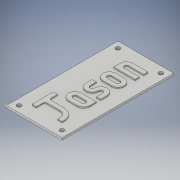
# Autodesk Inventor part: JASON
Saved by Autodesk Inventor 2017 (Build 210142000, 142)
## iProperties
Created: 2016-09-21
Part Number: JASON
Material: Generic
Document SubType Name: Modeling
Designer: vslabsal
Density: 1 g/cm^3
Appearance: Default
Author: vslabsal
Autodesk Inventor part; units mm, degrees
ref_plane "YZ Plane" through (0, 0, 0) normal (1, 0, 0) x (0, 1, 0)
ref_plane "XZ Plane" through (0, 0, 0) normal (0, 1, 0) x (-1, 0, 0)
ref_plane "XY Plane" through (0, 0, 0) normal (0, 0, 1) x (1, 0, 0)
sketch "Sketch1" plane through (0, 0, 0) normal (0, 1, 0) x (-1, 0, 0)
  line L0 (-82.55, -165.1) -> (0, -165.1)
  line L1 (0, -165.1) -> (0, 0)
  line L2 (0, 0) -> (-82.55, 0)
  line L3 (-82.55, 0) -> (-82.55, -165.1)
  circle A0 centre (-73.025, -155.575) radius 3.175
  circle A1 centre (-73.025, -155.575) radius 3.175
  circle A2 centre (-9.525, -155.575) radius 3.175
  circle A3 centre (-9.525, -155.575) radius 3.175
  circle A4 centre (-73.025, -9.525) radius 3.175
  circle A5 centre (-73.025, -9.525) radius 3.175
  circle A6 centre (-9.525, -9.525) radius 3.175
  circle A7 centre (-9.525, -9.525) radius 3.175
  constraints: 8 centre point, 8 end point, 2 coincident, 2 concentric, 2 parallel, 1 horizontal, 1 perpendicular
extrude "Extrusion1" add sketch "Sketch1" along normal blind 3.175
sketch "Sketch2" plane through (0, 3.175, 0) normal (0, 1, 0) x (1, 0, 0)
  line L0 (63.5, 19.05) -> (57.15, 19.05)
  line L1 (57.15, 19.05) -> (57.15, 22.225)
  line L2 (63.5, 19.05) -> (63.5, 22.225)
  arc A0 (57.15, 22.225) -> (47.625, 31.75) centre (47.625, 22.225) ccw
  arc A1 (63.5, 22.225) -> (47.625, 38.1) centre (47.625, 22.225) ccw
  line L3 (47.625, 31.75) -> (28.575, 31.75)
  line L4 (28.575, 38.1) -> (47.625, 38.1)
  arc A2 (28.575, 31.75) -> (25.4, 28.575) centre (28.575, 28.575) ccw
  arc A3 (25.4, 41.275) -> (28.575, 38.1) centre (28.575, 41.275) ccw
  line L5 (25.4, 19.05) -> (25.4, 28.575)
  line L6 (25.4, 19.05) -> (19.05, 19.05)
  line L7 (25.4, 41.275) -> (25.4, 50.8)
  line L8 (25.4, 50.8) -> (19.05, 50.8)
  line L9 (19.05, 50.8) -> (19.05, 19.05)
  point P0 (0, 0)
  constraints: 20 end point, 8 point on circle, 4 centre point, 3 perpendicular, 3 vertical, 2 horizontal, 1 coincident, 1 point on line
sketch "Sketch3" plane through (0, 3.175, 0) normal (0, 1, 0) x (1, 0, 0)
  point P0 (0, 0)
extrude "Extrusion2" add sketch "Sketch2" along normal blind 1.5875
sketch "Sketch4" plane through (0, 3.175, 0) normal (0, 1, 0) x (1, 0, 0)
  arc A0 (53.975, 57.15) -> (53.975, 63.5) centre (53.975, 60.325) ccw
  line L0 (53.975, 57.15) -> (41.275, 57.15)
  arc A1 (41.275, 63.5) -> (41.275, 57.15) centre (41.275, 60.325) ccw
  line L1 (41.275, 63.5) -> (53.975, 63.5)
  arc A2 (53.975, 50.8) -> (63.5, 60.325) centre (53.975, 60.325) ccw
  line L2 (53.975, 50.8) -> (41.275, 50.8)
  arc A3 (41.275, 69.85) -> (41.275, 50.8) centre (41.275, 60.325) ccw
  line L3 (41.275, 69.85) -> (63.5, 69.85)
  line L4 (63.5, 69.85) -> (63.5, 60.325)
  line L5 (57.15, 76.2) -> (63.5, 76.2)
  line L6 (63.5, 76.2) -> (63.5, 85.725)
  line L7 (57.15, 76.2) -> (57.15, 85.725)
  arc A4 (57.15, 85.725) -> (50.8, 85.725) centre (53.975, 85.725) ccw
  arc A5 (63.5, 85.725) -> (44.45, 85.725) centre (53.975, 85.725) ccw
  arc A6 (38.1, 85.725) -> (44.45, 85.725) centre (41.275, 85.725) ccw
  line L8 (31.75, 95.25) -> (38.1, 95.25)
  line L9 (38.1, 95.25) -> (38.1, 85.725)
  line L10 (41.275, 107.95) -> (53.975, 107.95)
  arc A7 (41.275, 114.3) -> (41.275, 107.95) centre (41.275, 111.125) ccw
  arc A8 (53.975, 107.95) -> (53.975, 114.3) centre (53.975, 111.125) ccw
  line L11 (53.975, 114.3) -> (41.275, 114.3)
  arc A9 (41.275, 120.65) -> (41.275, 101.6) centre (41.275, 111.125) ccw
  line L12 (41.275, 101.6) -> (53.975, 101.6)
  arc A10 (53.975, 101.6) -> (53.975, 120.65) centre (53.975, 111.125) ccw
  line L13 (53.975, 120.65) -> (41.275, 120.65)
  line L14 (63.5, 127) -> (63.5, 133.35)
  line L15 (63.5, 133.35) -> (41.275, 133.35)
  arc A11 (41.275, 139.7) -> (41.275, 133.35) centre (41.275, 136.525) ccw
  line L16 (41.275, 139.7) -> (63.5, 139.7)
  line L17 (63.5, 139.7) -> (63.5, 146.05)
  line L18 (63.5, 146.05) -> (41.275, 146.05)
  arc A12 (41.275, 146.05) -> (31.75, 136.525) centre (41.275, 136.525) ccw
  line L19 (63.5, 127) -> (31.75, 127)
  line L20 (31.75, 127) -> (31.75, 136.525)
  line L21 (57.15, 19.05) -> (57.15, 22.225) projected
  arc A13 (57.15, 22.225) -> (47.625, 31.75) centre (47.625, 22.225) ccw projected
  line L22 (47.625, 31.75) -> (28.575, 31.75) projected
  arc A14 (28.575, 31.75) -> (25.4, 28.575) centre (28.575, 28.575) ccw projected
  line L23 (25.4, 28.575) -> (25.4, 19.05) projected
  line L24 (25.4, 19.05) -> (19.05, 19.05) projected
  line L25 (19.05, 19.05) -> (19.05, 50.8) projected
  line L26 (19.05, 50.8) -> (25.4, 50.8) projected
  line L27 (25.4, 50.8) -> (25.4, 41.275) projected
  arc A15 (25.4, 41.275) -> (28.575, 38.1) centre (28.575, 41.275) ccw projected
  line L28 (28.575, 38.1) -> (47.625, 38.1) projected
  arc A16 (63.5, 22.225) -> (47.625, 38.1) centre (47.625, 22.225) ccw projected
  line L29 (63.5, 22.225) -> (63.5, 19.05) projected
  line L30 (63.5, 19.05) -> (57.15, 19.05) projected
  circle A17 centre (9.525, 9.525) radius 3.175 projected
  circle A18 centre (73.025, 9.525) radius 3.175 projected
  circle A19 centre (9.525, 155.575) radius 3.175 projected
  circle A20 centre (73.025, 155.575) radius 3.175 projected
  line L31 (82.55, 165.1) -> (0, 165.1) projected
  line L32 (0, 165.1) -> (0, 0) projected
  line L33 (0, 0) -> (82.55, 0) projected
  line L34 (82.55, 0) -> (82.55, 165.1) projected
  line L35 (31.75, 95.25) -> (31.75, 85.725)
  arc A21 (31.75, 85.725) -> (50.8, 85.725) centre (41.275, 85.725) ccw
  constraints: 44 end point, 28 point on circle, 14 centre point, 11 horizontal, 7 coincident, 7 perpendicular, 3 vertical, 1 tangent
extrude "Extrusion3" add sketch "Sketch4" along normal blind 1.5875 contours L2 A3 L3 L4 A2 | L7 A4 A21 L35 L8 L9 A6 A5 L6 L5 | L13 A10 L12 A9 | L19 L20 A12 L18 L17 L16 A11 L15 L14
body "Solid1"
